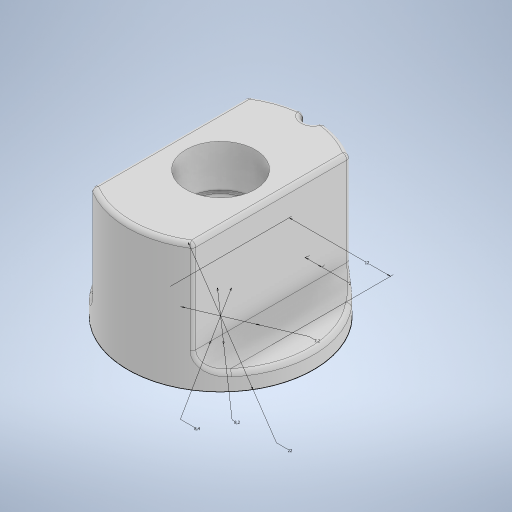
# Autodesk Inventor part: Switch4
Saved by Autodesk Inventor 2024 (Build 280153000, 153)
## iProperties
Created: 2023-06-19
Part Number: Switch4
Material: Типовые
Document SubType Name: Modeling
Designer: fm
Density: 1 g/cm^3
Appearance: По умолчанию
Author: fm
Autodesk Inventor part; units mm, degrees
ref_plane "YZ Plane" through (0, 0, 0) normal (1, 0, 0) x (0, 1, 0)
ref_plane "XZ Plane" through (0, 0, 0) normal (0, 1, 0) x (-1, 0, 0)
ref_plane "XY Plane" through (0, 0, 0) normal (0, 0, 1) x (1, 0, 0)
sketch "Эскиз1" plane through (0, 0, 0) normal (0, 1, 0) x (-1, 0, 0)
  circle A0 centre (0, 0) radius 4.1
  arc A1 (0.999, -10.9545) -> (-0.999, -10.9545) centre (0, 0) ccw
  line L0 (6, 0) -> (-6, 0) construction
  line L1 (6, -9.2195) -> (6, 9.2195)
  line L2 (-6, -9.2195) -> (-6, 9.2195)
  circle A2 centre (0, 0) radius 4
  arc A3 (0.999, -10.9545) -> (-0.999, -10.9545) centre (0, -11) ccw
  arc A4 (-1.0957, -3.4292) -> (-0.7657, -3.5176) centre (0, 0) ccw
  arc A5 (-2.2025, -2.8477) -> (-1.9226, -3.0436) centre (0, 0) ccw
  arc A6 (0.1433, -3.5971) -> (0.4836, -3.5674) centre (0, 0) ccw
  arc A7 (1.3649, -3.3312) -> (1.6745, -3.1868) centre (0, 0) ccw
  arc A8 (2.4219, -2.6635) -> (2.6635, -2.4219) centre (0, 0) ccw
  arc A9 (3.1868, -1.6745) -> (3.3312, -1.3649) centre (0, 0) ccw
  arc A10 (3.5674, -0.4836) -> (3.5971, -0.1433) centre (0, 0) ccw
  arc A11 (3.5176, 0.7657) -> (3.4292, 1.0957) centre (0, 0) ccw
  arc A12 (3.0436, 1.9226) -> (2.8477, 2.2025) centre (0, 0) ccw
  arc A13 (2.2025, 2.8477) -> (1.9226, 3.0436) centre (0, 0) ccw
  arc A14 (1.0957, 3.4292) -> (0.7657, 3.5176) centre (0, 0) ccw
  arc A15 (-0.1433, 3.5971) -> (-0.4836, 3.5674) centre (0, 0) ccw
  arc A16 (-1.3649, 3.3312) -> (-1.6745, 3.1868) centre (0, 0) ccw
  arc A17 (-2.4219, 2.6635) -> (-2.6635, 2.4219) centre (0, 0) ccw
  arc A18 (-3.1868, 1.6745) -> (-3.3312, 1.3649) centre (0, 0) ccw
  arc A19 (-3.5674, 0.4836) -> (-3.5971, 0.1433) centre (0, 0) ccw
  arc A20 (-3.5176, -0.7657) -> (-3.4292, -1.0957) centre (0, 0) ccw
  arc A21 (-3.0436, -1.9226) -> (-2.8477, -2.2025) centre (0, 0) ccw
  circle A22 centre (0, 0) radius 3.6
  arc A23 (-0.999, -10.9545) -> (0.999, -10.9545) centre (0, -11) ccw
  line L3 (0, 0) -> (0, -11) construction
  circle A24 centre (0, 0) radius 4.2
  point P0 (-3.5971, 0.1433)
  point P1 (-3.5176, -0.7657)
  point P2 (-3.4292, -1.0957)
  point P3 (-2.8477, -2.2025)
  point P4 (-2.2025, -2.8477)
  point P5 (-1.9226, -3.0436)
  point P6 (-1.0957, -3.4292)
  point P7 (-0.7657, -3.5176)
  point P8 (0.1433, -3.5971)
  point P9 (0.4836, -3.5674)
  point P10 (1.3649, -3.3312)
  point P11 (2.4219, -2.6635)
  point P12 (2.6635, -2.4219)
  point P13 (3.1868, -1.6745)
  point P14 (3.3312, -1.3649)
  point P15 (3.5674, -0.4836)
  point P16 (3.5971, -0.1433)
  point P17 (3.5176, 0.7657)
  point P18 (3.4292, 1.0957)
  point P19 (3.0436, 1.9226)
  point P20 (2.8477, 2.2025)
  point P21 (2.2025, 2.8477)
  point P22 (1.0957, 3.4292)
  point P23 (-0.1433, 3.5971)
  point P24 (-0.4836, 3.5674)
  point P25 (-1.3649, 3.3312)
  point P26 (-1.6745, 3.1868)
  point P27 (-2.4219, 2.6635)
  point P28 (-2.6635, 2.4219)
  point P29 (-3.3312, 1.3649)
  point P30 (-3.5674, 0.4836)
  dimension "d31" = 7.2
  dimension "d1" = 8.2
  dimension "d7" = 22
  dimension "d8" = 12
  dimension "d10" = 2
  dimension "d61" = 8.4
  constraints: 47 point on circle, 24 centre point, 8 coincident, 8 end point, 3 midpoint, 3 vertical, 1 horizontal, 20 other
  measures "d1" diameter of A0
  measures "d7" diameter of A1
  measures "d8" distance of L0.start L0.end
  measures "d10" diameter of A3
  measures "d61" diameter of A24
extrude "Выдавливание1" add sketch "Эскиз1" along normal blind 2 contours A0 | A3 A1 L2 L1 | L1 A1 | A1 L2 | A2 | A22 A5 A21 A20 A19 A18 A17 A16 A15 A14 A13 A12 A11 A10 A9 A8 A7 A6 A4 | A24
extrude "Выдавливание2" add sketch "Эскиз1" along normal blind 15 contours A0 | A3 A1 L2 L1 | A23 A3 | A2 | A22 A5 A21 A20 A19 A18 A17 A16 A15 A14 A13 A12 A11 A10 A9 A8 A7 A6 A4 | A24
fillet "Сопряжение3" radius 2 2 edges at (6, 2, 0) (-6, 2, 0)
fillet "Сопряжение7" radius 0.5 10 edges at (-6.6462, 2.5278, -8.7651) (-11, 2, 0) (-6.6462, 2.5278, 8.7651) (-6, 9.5, 9.2195) (-6, 9.5, -9.2195) (6.6464, 2.5276, 8.765) (11, 2, 0) (6.6464, 2.5276, -8.765) (6, 9.5, -9.2195) (6, 9.5, 9.2195)
extrude "Выдавливание10" cut sketch "Эскиз1" along normal blind 5 contours A0 | A2 | A22 A5 A21 A20 A19 A18 A17 A16 A15 A14 A13 A12 A11 A10 A9 A8 A7 A6 A4 | A24
extrude "Выдавливание11" cut sketch "Эскиз1" along normal through all contours A22 A5 A21 A20 A19 A18 A17 A16 A15 A14 A13 A12 A11 A10 A9 A8 A7 A6 A4
extrude "Выдавливание12" cut sketch "Эскиз1" against normal blind 5 from surface at 15 contours A0 | A2 | A22 A5 A21 A20 A19 A18 A17 A16 A15 A14 A13 A12 A11 A10 A9 A8 A7 A6 A4
extrude "Выдавливание13" cut sketch "Эскиз1" against normal blind 10 from surface at 15 contours A23 A3
fillet "Сопряжение14" radius 0.5 17 edges at (5.9364, 15, -9.1882) (6, 15, 0) (5.9364, 15, 9.1882) (0, 15, 11) (-5.9364, 15, 9.1882) (-6, 15, 0) (-5.9364, 15, -9.1882) (-3.472, 15, -10.4377) (3.472, 15, -10.4377) (0.999, 10, -10.9545) (0, 15, -10) (-0.999, 10, -10.9545) (0, 5, -10) (0, 5, -12) (-0.999, 2.5, -10.9545) (0.999, 1, -10.9545) (0.999, 3.5, -10.9545)
